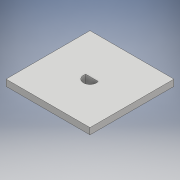
# Autodesk Inventor part: baseRotor1
Saved by Autodesk Inventor 2017 (Build 210142000, 142)
## iProperties
Created: 2017-08-06
Part Number: baseRotor1
Material: Generic
Document SubType Name: Sheet Metal
Designer: Bardo91
Density: 1 g/cm^3
Sheet Metal Rule: Default_mm
Appearance: Default
Author: Bardo91
Autodesk Inventor part; units mm, degrees
ref_plane "YZ Plane" through (0, 0, 0) normal (1, 0, 0) x (0, 1, 0)
ref_plane "XZ Plane" through (0, 0, 0) normal (0, 1, 0) x (-1, 0, 0)
ref_plane "XY Plane" through (0, 0, 0) normal (0, 0, 1) x (1, 0, 0)
sketch "Sketch8" plane through (0, 0, 0) normal (0, 0, 1) x (1, 0, 0)
  line L0 (0, 0) -> (40, 0)
  line L1 (40, 0) -> (40, 40)
  line L2 (40, 40) -> (0, 40)
  line L3 (0, 40) -> (0, 0)
  dimension "d35" = 40
  dimension "d36" = 40
  constraints: 8 end point, 2 parallel, 1 horizontal, 1 perpendicular
  measures "d35" distance of L2.end L1.end
  measures "d36" distance of L1.end L0.end
extrude "Extrusion8" add sketch "Sketch8" along normal blind 3
sketch "Sketch9" plane through (0, 0, 0) normal (0, 0, -1) x (-1, 0, 0)
  line L0 (0, 40) -> (0, 0) projected
  line L1 (0, 20) -> (-20, 20)
  circle A0 centre (-20, 20) radius 7.375
  dimension "d39" = 20
  dimension "d40" = 14.75
  constraints: 2 end point, 1 centre point, 1 coincident, 1 horizontal, 1 midpoint
  measures "d39" distance of L1.start L1.end
  measures "d40" diameter of A0
extrude "Extrusion9" add sketch "Sketch9" along normal blind 6
sketch "Sketch10" plane through (20, 20, -6) normal (0, 0, -1) x (-1, 0, 0)
  circle A0 centre (0, 0) radius 3.125
  line L0 (0, 0) -> (0, 1)
  line L1 (0, 1) -> (-2.9607, 1)
  line L2 (0, 1) -> (2.9607, 1)
  point P0 (20, -20)
  dimension "d43" = 6.25
  dimension "d44" = 1
  constraints: 6 end point, 2 point on circle, 1 centre point, 1 perpendicular, 1 point on line, 1 vertical
  measures "d43" diameter of A0
  measures "d44" distance of L0.start L0.end
extrude "Extrusion10" cut sketch "Sketch10" against normal up to next contours A0 L1 L2 picked at (-0.0807, -1.7325)
fillet "Fillet1" radius 0.5 2 edges at (20, 16.875, -6) (20, 21, -6)
equation "\"BendRadius\" = Thickness"
equation "\"BendReliefWidth\" = Thickness"
equation "\"BendReliefDepth\" = 0.5 * Thickness"
equation "\"CornerReliefSize\" = 4 * Thickness"
equation "\"MinimumRemnant\" = 2 * Thickness"
equation "\"TransitionRadius\" = BendRadius"
equation "\"JacobiRadiusSize\" = BendRadius"
equation "\"GapSize\" = Thickness"
equation "\"Thickness\" = 0.5"
body "Solid2"
